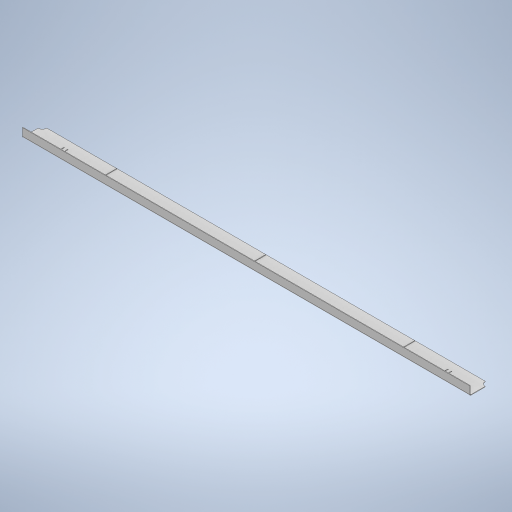
# Autodesk Inventor part: МОО 052 стрингер спина 22
Saved by Autodesk Inventor 2024.2 (Build 282272000, 272)
## iProperties
Created: 2024-04-28
Part Number: МОО 052 стрингер спина 22
Material: Stainless Steel
Document SubType Name: Sheet Metal
Designer: pokla
Density: 8 g/cm^3
Flat Pattern Width: 9.36541 cm
Flat Pattern Length: 150 cm
Flat Pattern Area: 1404.81 cm^2
Sheet Metal Rule: AISI304 2mm Die16
Sheet Metal Width: 93,654 mm
Sheet Metal Length: 1500,000 mm
Sheet Metal Area: 140481,176 mm^2
Appearance: Default
Author: admin
Autodesk Inventor part; units mm, degrees
ref_plane "YZ Plane" through (0, 0, 0) normal (1, 0, 0) x (0, 1, 0)
ref_plane "XZ Plane" through (0, 0, 0) normal (0, 1, 0) x (-1, 0, 0)
ref_plane "XY Plane" through (0, 0, 0) normal (0, 0, 1) x (1, 0, 0)
sketch "Sketch1" plane through (0, 0, 0) normal (0, 0, 1) x (1, 0, 0)
  line L0 (-750, 67.4521) -> (750, 67.4521)
  line L1 (750, 67.4521) -> (750, 0)
  line L2 (750, 0) -> (-750, 0)
  line L3 (-750, 0) -> (-750, 67.4521)
  point P0 (0, 0)
  point P1 (0, 0)
  dimension "d0" = 1500
  dimension "d1" = 67.4521
  measures "d0" distance of L1.end L2.end
  measures "d1" distance of L0.end L1.end
extrude "Plate1" add sketch "Sketch1" along normal blind 2
sketch "Sketch2" plane through (750, 2, 0) normal (0, -1, 0) x (1, 0, 0)
  line L0 (-1500, 0) -> (0, 0)
  line L1 (0, 0) -> (0, 30)
  line L2 (0, 30) -> (-1500, 30)
  line L3 (-1500, 30) -> (-1500, 0)
  constraints: 6 end point, 1 horizontal, 1 perpendicular, 1 vertical
edge flange "Flange1" height 30 angle 90 thickness 2 bend radius 2.75 thickness toward (0, -1, 0) relief round relief width 2 relief depth 1 edges at (0, 0, 2) wall of the first edge with corners at (-750, 2, 0) (750, 2, 0) (750, 2, 30) (-750, 2, 30)
bend "Bend1"
corner "Corner1"
sketch "Sketch5" plane through (0, 0, 0) normal (0, 0, -1) x (-1, 0, 0)
  line L0 (750, 67.4521) -> (-750, 67.4521) projected
  line L1 (-1, 30) -> (-1, 67.4521)
  line L2 (750, 0) -> (-750, 0) projected
  line L3 (-1, 30) -> (1, 30)
  line L4 (1, 30) -> (1, 67.4521)
  point P0 (0, 0)
  point P1 (0, 30)
  point P2 (0, 0)
  dimension "d27" = 2
  dimension "d29" = 30
  constraints: 6 end point, 2 midpoint, 2 point on line, 1 horizontal, 1 parallel, 1 perpendicular, 1 vertical alignment
  measures "d27" distance of L1.start L3.end
  measures "d29" distance from line of L2 L3.end
extrude "Extrusion1" cut sketch "Sketch5" against normal through all
pattern_linear "Rectangular Pattern1" count 3 spacing 500 along (1, 0, 0) of "Extrusion1" first direction both ways yes
sketch "Sketch6" plane through (0, 0, 0) normal (0, 0, -1) x (-1, 0, 0)
  line L0 (-750, 67.4521) -> (-750, 4.75) projected
  circle A0 centre (-750, 67.4521) radius 15
  line L1 (-750, 67.4521) -> (750, 67.4521) projected
  point P0 (0, 0)
  point P1 (-502, 51.9458)
  point P2 (-735, 67.4521)
  point P3 (-750, 52.4521)
  point P4 (750, 67.4521)
  dimension "d24" = 30
  constraints: 1 centre point, 1 other
  measures "d24" diameter of A0
extrude "Extrusion2" cut sketch "Sketch6" against normal through all contours L1 A0 L0 picked at (-740.1254, 66.3395)
mirror "Mirror1" about plane through (0, 0, 0) normal (1, 0, 0) of "Extrusion2"
sketch "Sketch7" plane through (0, 0, 2) normal (0, 0, 1) x (1, 0, 0)
  arc A0 (-750, 52.4521) -> (-735, 67.4521) centre (-750, 67.4521) ccw projected
  line L0 (-750, 4.75) -> (-750, 52.4521) projected
  line L1 (-750, 4.75) -> (750, 4.75) projected
  line L2 (750, 52.4521) -> (750, 4.75) projected
  arc A1 (735, 67.4521) -> (750, 52.4521) centre (750, 67.4521) ccw projected
  line L3 (501, 67.4521) -> (735, 67.4521) projected
  line L4 (501, 67.4521) -> (501, 30) projected
  line L5 (501, 30) -> (499, 30) projected
  line L6 (499, 30) -> (499, 67.4521) projected
  line L7 (1, 67.4521) -> (499, 67.4521) projected
  line L8 (1, 67.4521) -> (1, 30) projected
  line L9 (1, 30) -> (-1, 30) projected
  line L10 (-1, 30) -> (-1, 67.4521) projected
  line L11 (-499, 67.4521) -> (-1, 67.4521) projected
  line L12 (-499, 67.4521) -> (-499, 30) projected
  line L13 (-499, 30) -> (-501, 30) projected
  line L14 (-501, 30) -> (-501, 67.4521) projected
  line L15 (-735, 67.4521) -> (-501, 67.4521) projected
  line L16 (649, 32.1011) -> (651, 32.1011)
  line L17 (651, 32.1011) -> (651, 40.1011)
  line L18 (651, 40.1011) -> (649, 40.1011)
  line L19 (649, 40.1011) -> (649, 32.1011)
  line L20 (-750, 4.75) -> (750, 4.75) projected
  line L21 (650, 4.75) -> (650, 67.4521) construction
  line L22 (637, 32.1011) -> (639, 32.1011)
  line L23 (639, 32.1011) -> (639, 40.1011)
  line L24 (639, 40.1011) -> (637, 40.1011)
  line L25 (637, 40.1011) -> (637, 32.1011)
  point P0 (0, 0)
  point P1 (650, 32.1011)
  point P2 (649, 36.1011)
  point P3 (650, 36.1011)
  point P4 (639, 36.1011)
  dimension "d30" = 2
  dimension "d31" = 8
  dimension "d32" = 100
  dimension "d33" = 2
  dimension "d34" = 8
  dimension "d35" = 10
  constraints: 18 end point, 4 midpoint, 4 parallel, 3 perpendicular, 2 horizontal, 2 horizontal alignment, 2 point on line, 1 vertical alignment
  measures "d30" distance of L18.end L17.end
  measures "d31" distance of L17.end L16.end
  measures "d32" distance from line of L2 L21.end
  measures "d33" distance of L24.end L23.end
  measures "d34" distance of L23.end L22.end
  measures "d35" distance of L16.start L22.end
extrude "Extrusion3" cut sketch "Sketch7" along normal through all both and the other way through all contours L19 L18 L17 L16 | L25 L24 L23 L22
mirror "Mirror2" about plane through (0, 0, 0) normal (1, 0, 0) of "Extrusion3"
equation "\"d1\" = Стрингер_2"
equation "\"d27\" = d18"
equation "\"d29\" = Стрингер_глубина_паза"
equation "\"d2\" = Thickness"
equation "\"d3\" = BendReliefWidth"
equation "\"d4\" = BendReliefDepth"
equation "\"d5\" = MinimumRemnant"
equation "\"d6\" = TransitionRadius"
equation "\"d9\" = BendRadius"
equation "\"d10\" = CornerReliefSize"
equation "\"d11\" = GapSize"
equation "\"d12\" = JacobiRadiusSize"
equation "\"BendReliefWidth\" = Thickness"
equation "\"BendReliefDepth\" = 0.5 * Thickness"
equation "\"CornerReliefSize\" = 4 * Thickness"
equation "\"MinimumRemnant\" = 2 * Thickness"
equation "\"TransitionRadius\" = BendRadius"
equation "\"JacobiRadiusSize\" = BendRadius"
equation "\"GapSize\" = Thickness"
equation "\"d18\" = Thickness"
equation "\"qqqqqq\" = 67.35706"
equation "\"Стрингер_2\" = 67.452127"
equation "\"Стрингер_глубина_паза\" = 30"
equation "\"Thickness\" = 2"
equation "\"BendRadius\" = 2.75"
body "Solid1"
